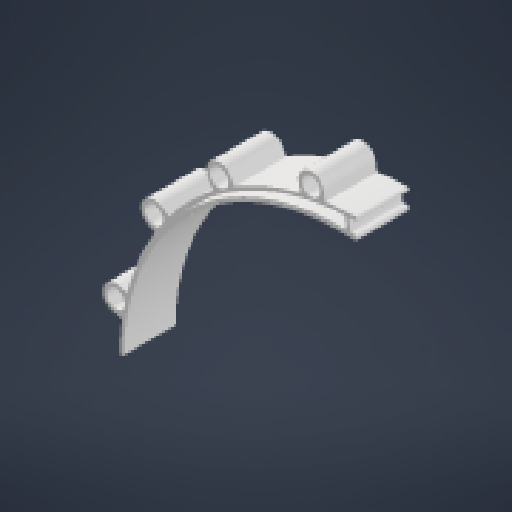
# Autodesk Inventor part: HalfFilterwall
Saved by Autodesk Inventor 2026 (Build 300175050, 175E)
## iProperties
Created: 2026-05-05
Part Number: HalfFilterwall
Material: Generic
Document SubType Name: Modeling
Designer: sniel
Density: 1 g/cm^3
Appearance: Default
Author: sniel
Autodesk Inventor part; units mm, degrees
ref_plane "YZ Plane" through (0, 0, 0) normal (1, 0, 0) x (0, 1, 0)
ref_plane "XZ Plane" through (0, 0, 0) normal (0, 1, 0) x (-1, 0, 0)
ref_plane "XY Plane" through (0, 0, 0) normal (0, 0, 1) x (1, 0, 0)
sketch "Sketch1" plane through (0, 0, 0) normal (0, 0, 1) x (1, 0, 0)
  line L0 (114.001828, -96.735526) -> (117.041325, -96.735526)
  arc A0 (117.041325, -96.735526) -> (-105.180629, -30.831618) centre (-9, -114.127341) ccw
  arc A1 (134.235526, -114.235526) -> (-105.180629, -30.831618) centre (0, -114.235526) ccw
  line L1 (134.235526, -114.235526) -> (136.235477, -114.235526)
  arc A2 (136.235477, -114.235526) -> (135.007021, -95.865294) centre (0, -114.119689) ccw
  line L2 (135.007021, -95.865294) -> (139.943419, -95.058908)
  arc A3 (139.943419, -95.058908) -> (137.133926, -80.329748) centre (138.734281, -87.657017) ccw
  line L3 (137.133926, -80.329748) -> (132.247295, -81.397042)
  arc A4 (132.247295, -81.397042) -> (116.651364, -43.745136) centre (0, -114.119689) ccw
  line L4 (116.651364, -43.745136) -> (120.861425, -41.044456)
  arc A5 (120.861425, -41.044456) -> (112.432948, -28.642756) centre (116.811886, -34.731673) ccw
  line L5 (112.432948, -28.642756) -> (108.372186, -31.563116)
  arc A6 (108.372186, -31.563116) -> (82.556573, -5.747503) centre (0, -114.119689) ccw
  line L6 (82.556573, -5.747503) -> (85.476933, -1.686741)
  arc A7 (85.476933, -1.686741) -> (73.075233, 6.741736) centre (79.388016, 2.692197) ccw
  line L7 (73.075233, 6.741736) -> (70.374553, 2.531675)
  arc A8 (70.374553, 2.531675) -> (32.722647, 18.127606) centre (0, -114.119689) ccw
  line L8 (32.722647, 18.127606) -> (33.789941, 23.014237)
  arc A9 (33.789941, 23.014237) -> (19.060781, 25.82373) centre (26.462672, 24.614592) ccw
  line L9 (19.060781, 25.82373) -> (18.254395, 20.887332)
  arc A10 (18.254395, 20.887332) -> (-18.254444, 20.887332) centre (-0.000025, -114.120055) ccw
  line L10 (-18.254444, 20.887332) -> (-19.060831, 25.82373)
  arc A11 (-19.060831, 25.82373) -> (-33.78999, 23.014237) centre (-26.462721, 24.614592) ccw
  line L11 (-33.78999, 23.014237) -> (-32.722696, 18.127606)
  arc A12 (-32.722696, 18.127606) -> (-70.374602, 2.531675) centre (-0.000049, -114.119689) ccw
  line L12 (-70.374602, 2.531675) -> (-73.075282, 6.741736)
  arc A13 (-73.075282, 6.741736) -> (-85.476982, -1.686741) centre (-79.388065, 2.692197) ccw
  line L13 (-85.476982, -1.686741) -> (-82.556623, -5.747503)
  arc A14 (-82.556623, -5.747503) -> (-108.372236, -31.563116) centre (-0.000049, -114.119689) ccw
  line L14 (-108.372236, -31.563116) -> (-112.432997, -28.642756)
  arc A15 (-112.432997, -28.642756) -> (-120.861475, -41.044456) centre (-116.811935, -34.731673) ccw
  line L15 (-120.861475, -41.044456) -> (-116.651414, -43.745136)
  arc A16 (-116.651414, -43.745136) -> (-132.247344, -81.397042) centre (-0.000049, -114.119689) ccw
  line L16 (-132.247344, -81.397042) -> (-137.133976, -80.329748)
  arc A17 (-137.133976, -80.329748) -> (-139.943468, -95.058908) centre (-138.734331, -87.657017) ccw
  line L17 (-139.943468, -95.058908) -> (-135.00707, -95.865294)
  arc A18 (-135.00707, -95.865294) -> (-136.235526, -114.235526) centre (-0.000049, -114.119689) ccw
  line L18 (-136.235526, -114.235526) -> (-134.235526, -114.235526)
  arc A19 (114.001828, -96.735526) -> (-134.235526, -114.235526) centre (-9.5, -114.235526) ccw
  circle A20 centre (138.734281, -87.772854) radius 5.25
  circle A21 centre (116.811886, -34.84751) radius 5.25
  circle A22 centre (26.462672, 24.498755) radius 5.25
  circle A23 centre (79.388016, 2.57636) radius 5.25
  circle A24 centre (-138.734281, -87.772854) radius 5.25
  circle A25 centre (-116.811886, -34.84751) radius 5.25
  circle A26 centre (-79.388016, 2.57636) radius 5.25
  circle A27 centre (-26.462672, 24.498755) radius 5.25
  line L19 (-0.000025, 22.115837) -> (-0.000025, 10.13771)
  line L20 (-3.753109, 13) -> (-5.751994, 13.066767)
  line L21 (-5.751994, 13.066767) -> (-7, 19.817361)
  line L22 (-7, 19.817361) -> (-5.002, 19.906773)
  line L23 (-5.002, 19.906773) -> (-3.753109, 13)
  point P0 (0, 0)
  point P1 (-0.000025, 12.789526)
  point P2 (-0.000025, 20)
  dimension "d2" = 2
  dimension "d3" = 2
  constraints: 48 end point, 46 point on circle, 28 centre point
  measures "d2" distance of L20.start L20.end
  measures "d3" distance of L21.end L22.end
extrude "Extrusion1" add sketch "Sketch1" along normal blind 30 contours A19 L18 A18 L17 A17 L16 A16 L15 A15 L14 A14 L13 A13 L12 A12 L11 A11 L10 A10 L19 A1 A0 L20 | L20 A0 | A0 L21 L22 L23 | L22 A1
fillet "Fillet1" radius 1 10 edges at (-136.2355, -114.2355, 15) (-134.2355, -114.2355, 15) (0, 20, 15) (0, 22.1158, 15) (0, 12.7895, 15) (0, 10.1377, 15) (-7, 19.8174, 15) (-5.002, 19.9068, 15) (-3.7531, 13, 15) (-5.752, 13.0668, 15)
sketch "Sketch2" plane through (0, 0, 30) normal (0, 0, 1) x (1, 0, 0)
  arc A0 (-1.067627, 10.214651) -> (-0.000025, 11.212363) centre (-1.000025, 11.212363) ccw
  line L0 (-0.000025, 11.212363) -> (-0.000025, 11.854483)
  arc A1 (-0.000025, 11.854483) -> (-0.936651, 12.852473) centre (-1.000025, 11.854483) ccw
  arc A2 (-0.936651, 12.852473) -> (-2.958612, 12.964721) centre (-9, -114.127341) ccw
  arc A3 (-3.895173, 13.785658) -> (-2.958612, 12.964721) centre (-2.91113, 13.963594) ccw
  line L1 (-3.895173, 13.785658) -> (-4.795999, 18.767522)
  arc A4 (-3.840567, 19.945048) -> (-4.795999, 18.767522) centre (-3.811957, 18.945458) ccw
  arc A5 (-0.99263, 19.99633) -> (-3.840567, 19.945048) centre (0, -114.235526) ccw
  arc A6 (-0.99263, 19.99633) -> (-0.000025, 20.996303) centre (-1.000025, 20.996303) ccw
  line L2 (-0.000025, 20.996303) -> (-0.000025, 21.11214)
  arc A7 (-0.000025, 21.11214) -> (-1.007419, 22.112112) centre (-1.000025, 21.11214) ccw
  arc A8 (-1.007419, 22.112112) -> (-18.254444, 20.887332) centre (-0.000025, -114.120055) ccw
  line L3 (-18.254444, 20.887332) -> (-19.060831, 25.82373)
  arc A9 (-19.060831, 25.82373) -> (-33.78999, 23.014237) centre (-26.462721, 24.614592) ccw
  line L4 (-33.78999, 23.014237) -> (-32.722696, 18.127606)
  arc A10 (-32.722696, 18.127606) -> (-70.374602, 2.531675) centre (-0.000049, -114.119689) ccw
  line L5 (-70.374602, 2.531675) -> (-73.075282, 6.741736)
  arc A11 (-73.075282, 6.741736) -> (-85.476982, -1.686741) centre (-79.388065, 2.692197) ccw
  line L6 (-85.476982, -1.686741) -> (-82.556623, -5.747503)
  arc A12 (-82.556623, -5.747503) -> (-108.372236, -31.563116) centre (-0.000049, -114.119689) ccw
  line L7 (-108.372236, -31.563116) -> (-112.432997, -28.642756)
  arc A13 (-112.432997, -28.642756) -> (-120.861475, -41.044456) centre (-116.811935, -34.731673) ccw
  line L8 (-120.861475, -41.044456) -> (-116.651414, -43.745136)
  arc A14 (-116.651414, -43.745136) -> (-132.247344, -81.397042) centre (-0.000049, -114.119689) ccw
  line L9 (-132.247344, -81.397042) -> (-137.133976, -80.329748)
  arc A15 (-137.133976, -80.329748) -> (-139.943468, -95.058908) centre (-138.734331, -87.657017) ccw
  line L10 (-139.943468, -95.058908) -> (-135.00707, -95.865294)
  arc A16 (-135.00707, -95.865294) -> (-136.232664, -113.228988) centre (-0.000049, -114.119689) ccw
  arc A17 (-136.232664, -113.228988) -> (-135.232685, -114.235526) centre (-135.232685, -113.235526) ccw
  line L11 (-135.232685, -114.235526) -> (-135.231549, -114.235526)
  arc A18 (-135.231549, -114.235526) -> (-134.231581, -113.243479) centre (-135.231549, -113.235526) ccw
  arc A19 (-1.067627, 10.214651) -> (-134.231581, -113.243479) centre (-9.5, -114.235526) ccw
  line L12 (-6.840001, 18.951909) -> (-5.975137, 14.273772)
  arc A20 (-6.974394, 13.092106) -> (-5.975137, 14.273772) centre (-6.958474, 14.091979) ccw
  arc A21 (-6.974394, 13.092106) -> (-105.180629, -30.831618) centre (-9, -114.127341) ccw
  arc A22 (-7.882056, 19.76839) -> (-105.180629, -30.831618) centre (0, -114.235526) ccw
  arc A23 (-6.840001, 18.951909) -> (-7.882056, 19.76839) centre (-7.823338, 18.770116) ccw
  circle A24 centre (-26.462672, 24.498755) radius 5.25
  circle A25 centre (-79.388016, 2.57636) radius 5.25
  circle A26 centre (-116.811886, -34.84751) radius 5.25
  circle A27 centre (-138.734281, -87.772854) radius 5.25
  circle A28 centre (0, -114.235526) radius 135.985526
  circle A29 centre (-116.811886, -34.84751) radius 5.25
  line L13 (-135.00707, -95.865294) -> (-133.577257, -88.756523)
  line L14 (-116.651414, -43.745136) -> (-112.46976, -37.798517)
  line L15 (-108.372236, -31.563116) -> (-112.46976, -37.798517)
  line L16 (-82.556623, -5.747503) -> (-76.437009, -1.765766)
  line L17 (-70.374602, 2.531675) -> (-76.437009, -1.765766)
  line L18 (-32.722696, 18.127606) -> (-25.479003, 19.341731)
  line L19 (-18.254444, 20.887332) -> (-25.479003, 19.341731)
  line L20 (-132.247344, -81.397042) -> (-133.577257, -88.756523)
  point P0 (0, 0)
  point P1 (-133.597973, -88.859519)
  point P2 (-112.46976, -37.798517)
  point P3 (-112.380148, -37.662149)
  point P4 (-76.61377, -1.880776)
  point P5 (-76.267979, -1.645946)
  point P6 (-25.711069, 19.302834)
  point P7 (-25.250255, 19.390669)
  point P8 (-112.566095, -37.935513)
  point P9 (-133.559143, -88.656284)
  constraints: 16 end point, 4 point on circle, 1 centre point, 1 coincident, 9 other
extrude "Extrusion2" cut sketch "Sketch2" against normal blind 20 contours L13 L10 A15 L9 L20 | L14 L8 A13 L7 L15 | L16 L6 A11 L5 L17 | L18 L4 A9 L3 L19
body "Solid1"
